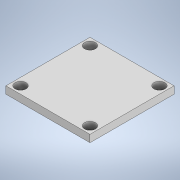
# Autodesk Inventor part: Mag_Sensor
Saved by Autodesk Inventor 2022 (Build 260153000, 153)
## iProperties
Created: 2022-03-24
Part Number: Mag_Sensor
Material: Generic
Document SubType Name: Modeling
Designer: Mlees
Density: 1 g/cm^3
Appearance: Default
Author: Mlees
Autodesk Inventor part; units mm, degrees
ref_plane "YZ Plane" through (0, 0, 0) normal (1, 0, 0) x (0, 1, 0)
ref_plane "XZ Plane" through (0, 0, 0) normal (0, 1, 0) x (-1, 0, 0)
ref_plane "XY Plane" through (0, 0, 0) normal (0, 0, 1) x (1, 0, 0)
sketch "Sketch1" plane through (0, 0, 0) normal (0, 1, 0) x (-1, 0, 0)
  line L0 (0, 0) -> (23, 0)
  line L1 (23, 0) -> (23, -23)
  line L2 (23, -23) -> (0, -23)
  line L3 (0, -23) -> (0, 0)
  line L4 (23, 0) -> (21, 0)
  circle A0 centre (21, -2) radius 1.5
  circle A1 centre (2, -2) radius 1.5
  circle A2 centre (21, -21) radius 1.5
  circle A3 centre (2, -21) radius 1.5
  dimension "d0" = 23
  dimension "d1" = 23
  dimension "d4" = 3
  constraints: 10 end point, 4 centre point, 2 parallel, 1 horizontal, 1 perpendicular, 1 point on line
  measures "d0" distance of L1.end L2.end
  measures "d1" distance of L0.end L1.end
  measures "d4" diameter of A0
extrude "Extrusion1" add sketch "Sketch1" along normal blind 2
body "Solid1"
